Autodesk Fusion 360 part; units mm, degrees
(part 2 of 5)
  spline S268 degree 3 poles (57.7936, -18.906) (57.5187, -18.906) (57.2937, -18.681) (57.2937, -18.406) knots 0 0 0 0 1 1 1 1
  line L268 (57.2937, -18.406) -> (57.2937, -5.4062)
  spline S269 degree 3 poles (57.2937, -5.4062) (57.2937, -5.1311) (57.5187, -4.9062) (57.7936, -4.9062) knots 2 2 2 2 3 3 3 3
  line L269 (57.7936, -4.9062) -> (70.7933, -4.9062)
  spline S270 degree 3 poles (70.7933, -4.9062) (71.0686, -4.9062) (71.2935, -5.1311) (71.2935, -5.4062) knots 4 4 4 4 5 5 5 5
  line L270 (71.2935, -5.4062) -> (71.2935, -18.406)
  spline S271 degree 3 poles (71.2935, -18.406) (71.2935, -18.681) (71.0686, -18.906) (70.7933, -18.906) knots 6 6 6 6 7 7 7 7
  line L271 (70.7933, -18.906) -> (57.7936, -18.906)
  spline S272 degree 3 poles (-57.0067, -5.4062) (-57.0067, -5.1311) (-56.7818, -4.9062) (-56.5068, -4.9062) knots 0 0 0 0 1 1 1 1
  line L272 (-56.5068, -4.9062) -> (-43.5068, -4.9062)
  spline S273 degree 3 poles (-43.5068, -4.9062) (-43.2315, -4.9062) (-43.0065, -5.1311) (-43.0065, -5.4062) knots 2 2 2 2 3 3 3 3
  line L273 (-43.0065, -5.4062) -> (-43.0065, -18.406)
  spline S274 degree 3 poles (-43.0065, -18.406) (-43.0065, -18.681) (-43.2315, -18.906) (-43.5068, -18.906) knots 4 4 4 4 5 5 5 5
  line L274 (-43.5068, -18.906) -> (-56.5068, -18.906)
  spline S275 degree 3 poles (-56.5068, -18.906) (-56.7818, -18.906) (-57.0067, -18.681) (-57.0067, -18.406) knots 6 6 6 6 7 7 7 7
  line L275 (-57.0067, -18.406) -> (-57.0067, -5.4062)
  spline S276 degree 3 poles (129.2304, 0.144) (128.9555, 0.144) (128.7306, 0.369) (128.7306, 0.6441) knots 0 0 0 0 1 1 1 1
  line L276 (128.7306, 0.6441) -> (128.7306, 13.6438)
  spline S277 degree 3 poles (128.7306, 13.6438) (128.7306, 13.9189) (128.9555, 14.1438) (129.2304, 14.1438) knots 2 2 2 2 3 3 3 3
  line L277 (129.2304, 14.1438) -> (142.2305, 14.1438)
  spline S278 degree 3 poles (142.2305, 14.1438) (142.5058, 14.1438) (142.7307, 13.9189) (142.7307, 13.6438) knots 4 4 4 4 5 5 5 5
  line L278 (142.7307, 13.6438) -> (142.7307, 0.6441)
  spline S279 degree 3 poles (142.7307, 0.6441) (142.7307, 0.369) (142.5058, 0.144) (142.2305, 0.144) knots 6 6 6 6 7 7 7 7
  line L279 (142.2305, 0.144) -> (129.2304, 0.144)
  spline S280 degree 3 poles (76.8436, -18.906) (76.5687, -18.906) (76.3437, -18.681) (76.3437, -18.406) knots 0 0 0 0 1 1 1 1
  line L280 (76.3437, -18.406) -> (76.3437, -5.4062)
  spline S281 degree 3 poles (76.3437, -5.4062) (76.3437, -5.1311) (76.5687, -4.9062) (76.8436, -4.9062) knots 2 2 2 2 3 3 3 3
  line L281 (76.8436, -4.9062) -> (89.8433, -4.9062)
  spline S282 degree 3 poles (89.8433, -4.9062) (90.1186, -4.9062) (90.3436, -5.1311) (90.3436, -5.4062) knots 4 4 4 4 5 5 5 5
  line L282 (90.3436, -5.4062) -> (90.3436, -18.406)
  spline S283 degree 3 poles (90.3436, -18.406) (90.3436, -18.681) (90.1186, -18.906) (89.8433, -18.906) knots 6 6 6 6 7 7 7 7
  line L283 (89.8433, -18.906) -> (76.8436, -18.906)
  spline S284 degree 3 poles (23.9555, 32.6938) (23.9555, 32.9689) (24.1805, 33.1939) (24.4554, 33.1939) knots 0 0 0 0 1 1 1 1
  line L284 (24.4554, 33.1939) -> (37.4554, 33.1939)
  spline S285 degree 3 poles (37.4554, 33.1939) (37.7307, 33.1939) (37.9557, 32.9689) (37.9557, 32.6938) knots 2 2 2 2 3 3 3 3
  line L285 (37.9557, 32.6938) -> (37.9557, 19.6941)
  spline S286 degree 3 poles (37.9557, 19.6941) (37.9557, 19.419) (37.7307, 19.194) (37.4554, 19.194) knots 4 4 4 4 5 5 5 5
  line L286 (37.4554, 19.194) -> (24.4554, 19.194)
  spline S287 degree 3 poles (24.4554, 19.194) (24.1805, 19.194) (23.9555, 19.419) (23.9555, 19.6941) knots 6 6 6 6 7 7 7 7
  line L287 (23.9555, 19.6941) -> (23.9555, 32.6938)
  spline S288 degree 3 poles (95.3937, -5.4062) (95.3937, -5.1311) (95.6187, -4.9062) (95.8936, -4.9062) knots 0 0 0 0 1 1 1 1
  line L288 (95.8936, -4.9062) -> (108.8933, -4.9062)
  spline S289 degree 3 poles (108.8933, -4.9062) (109.1686, -4.9062) (109.3936, -5.1311) (109.3936, -5.4062) knots 2 2 2 2 3 3 3 3
  line L289 (109.3936, -5.4062) -> (109.3936, -18.406)
  spline S290 degree 3 poles (109.3936, -18.406) (109.3936, -18.681) (109.1686, -18.906) (108.8933, -18.906) knots 4 4 4 4 5 5 5 5
  line L290 (108.8933, -18.906) -> (95.8936, -18.906)
  spline S291 degree 3 poles (95.8936, -18.906) (95.6187, -18.906) (95.3937, -18.681) (95.3937, -18.406) knots 6 6 6 6 7 7 7 7
  line L291 (95.3937, -18.406) -> (95.3937, -5.4062)
  spline S292 degree 3 poles (38.7436, -18.906) (38.4687, -18.906) (38.2437, -18.681) (38.2437, -18.406) knots 0 0 0 0 1 1 1 1
  line L292 (38.2437, -18.406) -> (38.2437, -5.4062)
  spline S293 degree 3 poles (38.2437, -5.4062) (38.2437, -5.1311) (38.4687, -4.9062) (38.7436, -4.9062) knots 2 2 2 2 3 3 3 3
  line L293 (38.7436, -4.9062) -> (51.7433, -4.9062)
  spline S294 degree 3 poles (51.7433, -4.9062) (52.0186, -4.9062) (52.2435, -5.1311) (52.2435, -5.4062) knots 4 4 4 4 5 5 5 5
  line L294 (52.2435, -5.4062) -> (52.2435, -18.406)
  spline S295 degree 3 poles (52.2435, -18.406) (52.2435, -18.681) (52.0186, -18.906) (51.7433, -18.906) knots 6 6 6 6 7 7 7 7
  line L295 (51.7433, -18.906) -> (38.7436, -18.906)
  spline S296 degree 3 poles (-14.1445, 56.506) (-14.1445, 56.7811) (-13.9196, 57.006) (-13.6447, 57.006) knots 0 0 0 0 1 1 1 1
  line L296 (-13.6447, 57.006) -> (-0.6446, 57.006)
  spline S297 degree 3 poles (-0.6446, 57.006) (-0.3693, 57.006) (-0.1443, 56.7811) (-0.1443, 56.506) knots 2 2 2 2 3 3 3 3
  line L297 (-0.1443, 56.506) -> (-0.1443, 43.5059)
  spline S298 degree 3 poles (-0.1443, 43.5059) (-0.1443, 43.2308) (-0.3693, 43.0058) (-0.6446, 43.0058) knots 4 4 4 4 5 5 5 5
  line L298 (-0.6446, 43.0058) -> (-13.6447, 43.0058)
  spline S299 degree 3 poles (-13.6447, 43.0058) (-13.9196, 43.0058) (-14.1445, 43.2308) (-14.1445, 43.5059) knots 6 6 6 6 7 7 7 7
  line L299 (-14.1445, 43.5059) -> (-14.1445, 56.506)
  spline S300 degree 3 poles (91.1304, 0.144) (90.8555, 0.144) (90.6305, 0.369) (90.6305, 0.6441) knots 0 0 0 0 1 1 1 1
  line L300 (90.6305, 0.6441) -> (90.6305, 13.6438)
  spline S301 degree 3 poles (90.6305, 13.6438) (90.6305, 13.9189) (90.8555, 14.1438) (91.1304, 14.1438) knots 2 2 2 2 3 3 3 3
  line L301 (91.1304, 14.1438) -> (104.1305, 14.1438)
  spline S302 degree 3 poles (104.1305, 14.1438) (104.4058, 14.1438) (104.6307, 13.9189) (104.6307, 13.6438) knots 4 4 4 4 5 5 5 5
  line L302 (104.6307, 13.6438) -> (104.6307, 0.6441)
  spline S303 degree 3 poles (104.6307, 0.6441) (104.6307, 0.369) (104.4058, 0.144) (104.1305, 0.144) knots 6 6 6 6 7 7 7 7
  line L303 (104.1305, 0.144) -> (91.1304, 0.144)
  spline S304 degree 3 poles (-23.1697, 0.144) (-23.4446, 0.144) (-23.6695, 0.369) (-23.6695, 0.6441) knots 0 0 0 0 1 1 1 1
  line L304 (-23.6695, 0.6441) -> (-23.6695, 13.6438)
  spline S305 degree 3 poles (-23.6695, 13.6438) (-23.6695, 13.9189) (-23.4446, 14.1438) (-23.1697, 14.1438) knots 2 2 2 2 3 3 3 3
  line L305 (-23.1697, 14.1438) -> (-10.1696, 14.1438)
  spline S306 degree 3 poles (-10.1696, 14.1438) (-9.8943, 14.1438) (-9.6694, 13.9189) (-9.6694, 13.6438) knots 4 4 4 4 5 5 5 5
  line L306 (-9.6694, 13.6438) -> (-9.6694, 0.6441)
  spline S307 degree 3 poles (-9.6694, 0.6441) (-9.6694, 0.369) (-9.8943, 0.144) (-10.1696, 0.144) knots 6 6 6 6 7 7 7 7
  line L307 (-10.1696, 0.144) -> (-23.1697, 0.144)
  spline S308 degree 3 poles (-61.2697, 0.144) (-61.5446, 0.144) (-61.7696, 0.369) (-61.7696, 0.6441) knots 0 0 0 0 1 1 1 1
  line L308 (-61.7696, 0.6441) -> (-61.7696, 13.6438)
  spline S309 degree 3 poles (-61.7696, 13.6438) (-61.7696, 13.9189) (-61.5446, 14.1438) (-61.2697, 14.1438) knots 2 2 2 2 3 3 3 3
  line L309 (-61.2697, 14.1438) -> (-48.2696, 14.1438)
  spline S310 degree 3 poles (-48.2696, 14.1438) (-47.9943, 14.1438) (-47.7694, 13.9189) (-47.7694, 13.6438) knots 4 4 4 4 5 5 5 5
  line L310 (-47.7694, 13.6438) -> (-47.7694, 0.6441)
  spline S311 degree 3 poles (-47.7694, 0.6441) (-47.7694, 0.369) (-47.9943, 0.144) (-48.2696, 0.144) knots 6 6 6 6 7 7 7 7
  line L311 (-48.2696, 0.144) -> (-61.2697, 0.144)
  spline S312 degree 3 poles (119.2056, 32.6938) (119.2056, 32.9689) (119.4305, 33.1939) (119.7054, 33.1939) knots 0 0 0 0 1 1 1 1
  line L312 (119.7054, 33.1939) -> (132.7055, 33.1939)
  spline S313 degree 3 poles (132.7055, 33.1939) (132.9808, 33.1939) (133.2057, 32.9689) (133.2057, 32.6938) knots 2 2 2 2 3 3 3 3
  line L313 (133.2057, 32.6938) -> (133.2057, 19.6941)
  spline S314 degree 3 poles (133.2057, 19.6941) (133.2057, 19.419) (132.9808, 19.194) (132.7055, 19.194) knots 4 4 4 4 5 5 5 5
  line L314 (132.7055, 19.194) -> (119.7054, 19.194)
  spline S315 degree 3 poles (119.7054, 19.194) (119.4305, 19.194) (119.2056, 19.419) (119.2056, 19.6941) knots 6 6 6 6 7 7 7 7
  line L315 (119.2056, 19.6941) -> (119.2056, 32.6938)
  spline S316 degree 3 poles (4.9055, 32.6938) (4.9055, 32.9689) (5.1304, 33.1939) (5.4054, 33.1939) knots 0 0 0 0 1 1 1 1
  line L316 (5.4054, 33.1939) -> (18.4054, 33.1939)
  spline S317 degree 3 poles (18.4054, 33.1939) (18.6807, 33.1939) (18.9057, 32.9689) (18.9057, 32.6938) knots 2 2 2 2 3 3 3 3
  line L317 (18.9057, 32.6938) -> (18.9057, 19.6941)
  spline S318 degree 3 poles (18.9057, 19.6941) (18.9057, 19.419) (18.6807, 19.194) (18.4054, 19.194) knots 4 4 4 4 5 5 5 5
  line L318 (18.4054, 19.194) -> (5.4054, 19.194)
  spline S319 degree 3 poles (5.4054, 19.194) (5.1304, 19.194) (4.9055, 19.419) (4.9055, 19.6941) knots 6 6 6 6 7 7 7 7
  line L319 (4.9055, 19.6941) -> (4.9055, 32.6938)
  line L320 (71.5805, 0.6441) -> (71.5805, 13.6438)
  spline S320 degree 3 poles (71.5805, 13.6438) (71.5805, 13.9189) (71.8055, 14.1438) (72.0804, 14.1438) knots 1 1 1 1 2 2 2 2
  line L321 (72.0804, 14.1438) -> (85.0805, 14.1438)
  spline S321 degree 3 poles (85.0805, 14.1438) (85.3557, 14.1438) (85.5807, 13.9189) (85.5807, 13.6438) knots 3 3 3 3 4 4 4 4
  line L322 (85.5807, 13.6438) -> (85.5807, 0.6441)
  spline S322 degree 3 poles (85.5807, 0.6441) (85.5807, 0.369) (85.3557, 0.144) (85.0805, 0.144) knots 5 5 5 5 6 6 6 6
  line L323 (85.0805, 0.144) -> (72.0804, 0.144)
  spline S323 degree 3 poles (72.0804, 0.144) (71.8055, 0.144) (71.5805, 0.369) (71.5805, 0.6441) knots 7 7 7 7 8 8 8 8
  spline S324 degree 3 poles (81.1055, 56.506) (81.1055, 56.7811) (81.3305, 57.006) (81.6054, 57.006) knots 0 0 0 0 1 1 1 1
  line L324 (81.6054, 57.006) -> (94.6055, 57.006)
  spline S325 degree 3 poles (94.6055, 57.006) (94.8807, 57.006) (95.1057, 56.7811) (95.1057, 56.506) knots 2 2 2 2 3 3 3 3
  line L325 (95.1057, 56.506) -> (95.1057, 43.5059)
  spline S326 degree 3 poles (95.1057, 43.5059) (95.1057, 43.2308) (94.8807, 43.0058) (94.6055, 43.0058) knots 4 4 4 4 5 5 5 5
  line L326 (94.6055, 43.0058) -> (81.6054, 43.0058)
  spline S327 degree 3 poles (81.6054, 43.0058) (81.3305, 43.0058) (81.1055, 43.2308) (81.1055, 43.5059) knots 6 6 6 6 7 7 7 7
  line L327 (81.1055, 43.5059) -> (81.1055, 56.506)
  spline S328 degree 3 poles (66.8187, -24.4562) (66.8187, -24.1811) (67.0437, -23.9562) (67.3186, -23.9562) knots 0 0 0 0 1 1 1 1
  line L328 (67.3186, -23.9562) -> (80.3183, -23.9562)
  spline S329 degree 3 poles (80.3183, -23.9562) (80.5936, -23.9562) (80.8185, -24.1811) (80.8185, -24.4562) knots 2 2 2 2 3 3 3 3
  line L329 (80.8185, -24.4562) -> (80.8185, -37.456)
  spline S330 degree 3 poles (80.8185, -37.456) (80.8185, -37.7311) (80.5936, -37.956) (80.3183, -37.956) knots 4 4 4 4 5 5 5 5
  line L330 (80.3183, -37.956) -> (67.3186, -37.956)
  spline S331 degree 3 poles (67.3186, -37.956) (67.0437, -37.956) (66.8187, -37.7311) (66.8187, -37.456) knots 6 6 6 6 7 7 7 7
  line L331 (66.8187, -37.456) -> (66.8187, -24.4562)
  spline S332 degree 3 poles (9.6687, -24.4562) (9.6687, -24.1811) (9.8936, -23.9562) (10.1686, -23.9562) knots 0 0 0 0 1 1 1 1
  line L332 (10.1686, -23.9562) -> (23.1683, -23.9562)
  spline S333 degree 3 poles (23.1683, -23.9562) (23.4435, -23.9562) (23.6685, -24.1811) (23.6685, -24.4562) knots 2 2 2 2 3 3 3 3
  line L333 (23.6685, -24.4562) -> (23.6685, -37.456)
  spline S334 degree 3 poles (23.6685, -37.456) (23.6685, -37.7311) (23.4435, -37.956) (23.1683, -37.956) knots 4 4 4 4 5 5 5 5
  line L334 (23.1683, -37.956) -> (10.1686, -37.956)
  spline S335 degree 3 poles (10.1686, -37.956) (9.8936, -37.956) (9.6687, -37.7311) (9.6687, -37.456) knots 6 6 6 6 7 7 7 7
  line L335 (9.6687, -37.456) -> (9.6687, -24.4562)
  spline S336 degree 3 poles (62.0555, 32.6938) (62.0555, 32.9689) (62.2805, 33.1939) (62.5554, 33.1939) knots 0 0 0 0 1 1 1 1
  line L336 (62.5554, 33.1939) -> (75.5555, 33.1939)
  spline S337 degree 3 poles (75.5555, 33.1939) (75.8307, 33.1939) (76.0557, 32.9689) (76.0557, 32.6938) knots 2 2 2 2 3 3 3 3
  line L337 (76.0557, 32.6938) -> (76.0557, 19.6941)
  spline S338 degree 3 poles (76.0557, 19.6941) (76.0557, 19.419) (75.8307, 19.194) (75.5555, 19.194) knots 4 4 4 4 5 5 5 5
  line L338 (75.5555, 19.194) -> (62.5554, 19.194)
  spline S339 degree 3 poles (62.5554, 19.194) (62.2805, 19.194) (62.0555, 19.419) (62.0555, 19.6941) knots 6 6 6 6 7 7 7 7
  line L339 (62.0555, 19.6941) -> (62.0555, 32.6938)
  spline S340 degree 3 poles (43.0055, 56.506) (43.0055, 56.7811) (43.2305, 57.006) (43.5054, 57.006) knots 0 0 0 0 1 1 1 1
  line L340 (43.5054, 57.006) -> (56.5055, 57.006)
  spline S341 degree 3 poles (56.5055, 57.006) (56.7807, 57.006) (57.0057, 56.7811) (57.0057, 56.506) knots 2 2 2 2 3 3 3 3
  line L341 (57.0057, 56.506) -> (57.0057, 43.5059)
  spline S342 degree 3 poles (57.0057, 43.5059) (57.0057, 43.2308) (56.7807, 43.0058) (56.5055, 43.0058) knots 4 4 4 4 5 5 5 5
  line L342 (56.5055, 43.0058) -> (43.5054, 43.0058)
  spline S343 degree 3 poles (43.5054, 43.0058) (43.2305, 43.0058) (43.0055, 43.2308) (43.0055, 43.5059) knots 6 6 6 6 7 7 7 7
  line L343 (43.0055, 43.5059) -> (43.0055, 56.506)
  spline S344 degree 3 poles (-52.2446, 32.6938) (-52.2446, 32.9689) (-52.0196, 33.1939) (-51.7447, 33.1939) knots 0 0 0 0 1 1 1 1
  line L344 (-51.7447, 33.1939) -> (-38.7446, 33.1939)
  spline S345 degree 3 poles (-38.7446, 33.1939) (-38.4693, 33.1939) (-38.2444, 32.9689) (-38.2444, 32.6938) knots 2 2 2 2 3 3 3 3
  line L345 (-38.2444, 32.6938) -> (-38.2444, 19.6941)
  spline S346 degree 3 poles (-38.2444, 19.6941) (-38.2444, 19.419) (-38.4693, 19.194) (-38.7446, 19.194) knots 4 4 4 4 5 5 5 5
  line L346 (-38.7446, 19.194) -> (-51.7447, 19.194)
  spline S347 degree 3 poles (-51.7447, 19.194) (-52.0196, 19.194) (-52.2446, 19.419) (-52.2446, 19.6941) knots 6 6 6 6 7 7 7 7
  line L347 (-52.2446, 19.6941) -> (-52.2446, 32.6938)
  spline S348 degree 3 poles (81.1055, 32.6938) (81.1055, 32.9689) (81.3305, 33.1939) (81.6054, 33.1939) knots 0 0 0 0 1 1 1 1
  line L348 (81.6054, 33.1939) -> (94.6055, 33.1939)
  spline S349 degree 3 poles (94.6055, 33.1939) (94.8807, 33.1939) (95.1057, 32.9689) (95.1057, 32.6938) knots 2 2 2 2 3 3 3 3
  line L349 (95.1057, 32.6938) -> (95.1057, 19.6941)
  spline S350 degree 3 poles (95.1057, 19.6941) (95.1057, 19.419) (94.8807, 19.194) (94.6055, 19.194) knots 4 4 4 4 5 5 5 5
  line L350 (94.6055, 19.194) -> (81.6054, 19.194)
  spline S351 degree 3 poles (81.6054, 19.194) (81.3305, 19.194) (81.1055, 19.419) (81.1055, 19.6941) knots 6 6 6 6 7 7 7 7
  line L351 (81.1055, 19.6941) -> (81.1055, 32.6938)
  spline S352 degree 3 poles (-100.1566, -56.506) (-100.1566, -56.7811) (-100.3815, -57.006) (-100.6568, -57.006) knots 0 0 0 0 1 1 1 1
  line L352 (-100.6568, -57.006) -> (-113.6569, -57.006)
  spline S353 degree 3 poles (-113.6569, -57.006) (-113.9318, -57.006) (-114.1568, -56.7811) (-114.1568, -56.506) knots 2 2 2 2 3 3 3 3
  line L353 (-114.1568, -56.506) -> (-114.1568, -43.5062)
  spline S354 degree 3 poles (-114.1568, -43.5062) (-114.1568, -43.2312) (-113.9318, -43.0062) (-113.6569, -43.0062) knots 4 4 4 4 5 5 5 5
  line L354 (-113.6569, -43.0062) -> (-100.6568, -43.0062)
  spline S355 degree 3 poles (-100.6568, -43.0062) (-100.3815, -43.0062) (-100.1566, -43.2312) (-100.1566, -43.5062) knots 6 6 6 6 7 7 7 7
  line L355 (-100.1566, -43.5062) -> (-100.1566, -56.506)
  spline S356 degree 3 poles (99.8686, -37.456) (99.8686, -37.7311) (99.6436, -37.956) (99.3683, -37.956) knots 0 0 0 0 1 1 1 1
  line L356 (99.3683, -37.956) -> (86.3686, -37.956)
  spline S357 degree 3 poles (86.3686, -37.956) (86.0937, -37.956) (85.8687, -37.7311) (85.8687, -37.456) knots 2 2 2 2 3 3 3 3
  line L357 (85.8687, -37.456) -> (85.8687, -24.4562)
  spline S358 degree 3 poles (85.8687, -24.4562) (85.8687, -24.1811) (86.0937, -23.9562) (86.3686, -23.9562) knots 4 4 4 4 5 5 5 5
  line L358 (86.3686, -23.9562) -> (99.3683, -23.9562)
  spline S359 degree 3 poles (99.3683, -23.9562) (99.6436, -23.9562) (99.8686, -24.1811) (99.8686, -24.4562) knots 6 6 6 6 7 7 7 7
  line L359 (99.8686, -24.4562) -> (99.8686, -37.456)
  spline S360 degree 3 poles (-55.3386, -30.9561) (-55.3386, -31.2312) (-55.4681, -31.4562) (-55.6263, -31.4562) (-55.7847, -31.4562) (-55.9143, -31.6811) (-55.9143, -31.9562) knots 0 0 0 0 1 1 1 2 2 2 2
  line L360 (-55.9143, -31.9562) -> (-55.9143, -37.2262)
  spline S361 degree 3 poles (-55.9143, -37.2262) (-55.9143, -37.5013) (-56.1392, -37.7262) (-56.4142, -37.7262) knots 3 3 3 3 4 4 4 4
  line L361 (-56.4142, -37.7262) -> (-57.139, -37.7262)
  spline S362 degree 3 poles (-57.139, -37.7262) (-57.4143, -37.7262) (-57.6392, -37.9512) (-57.6392, -38.2263) knots 5 5 5 5 6 6 6 6
  line L362 (-57.6392, -38.2263) -> (-57.6392, -38.4261)
  spline S363 degree 3 poles (-57.6392, -38.4261) (-57.6392, -38.7012) (-57.8642, -38.9262) (-58.1391, -38.9262) knots 7 7 7 7 8 8 8 8
  line L363 (-58.1391, -38.9262) -> (-60.7891, -38.9262)
  spline S364 degree 3 poles (-60.7891, -38.9262) (-61.064, -38.9262) (-61.289, -38.7012) (-61.289, -38.4261) knots 9 9 9 9 10 10 10 10
  line L364 (-61.289, -38.4261) -> (-61.289, -38.2263)
  spline S365 degree 3 poles (-61.289, -38.2263) (-61.289, -37.9512) (-61.5139, -37.7262) (-61.7892, -37.7262) knots 11 11 11 11 12 12 12 12
  line L365 (-61.7892, -37.7262) -> (-62.5141, -37.7262)
  spline S366 degree 3 poles (-62.5141, -37.7262) (-62.7893, -37.7262) (-63.0143, -37.5013) (-63.0143, -37.2262) knots 13 13 13 13 14 14 14 14
  line L366 (-63.0143, -37.2262) -> (-63.0143, -33.7563)
  spline S367 degree 3 poles (-63.0143, -33.7563) (-63.0143, -33.4812) (-63.2392, -33.2562) (-63.5142, -33.2562) knots 15 15 15 15 16 16 16 16
  line L367 (-63.5142, -33.2562) -> (-63.9386, -33.2562)
  spline S368 degree 3 poles (-63.9386, -33.2562) (-64.2135, -33.2562) (-64.4385, -33.4812) (-64.4385, -33.7563) knots 17 17 17 17 18 18 18 18
  line L368 (-64.4385, -33.7563) -> (-64.4385, -37.456)
  spline S369 degree 3 poles (-64.4385, -37.456) (-64.4385, -37.7311) (-64.6635, -37.956) (-64.9387, -37.956) knots 19 19 19 19 20 20 20 20
  line L369 (-64.9387, -37.956) -> (-77.9388, -37.956)
  spline S370 degree 3 poles (-77.9388, -37.956) (-78.2137, -37.956) (-78.4387, -37.7311) (-78.4387, -37.456) knots 21 21 21 21 22 22 22 22
  line L370 (-78.4387, -37.456) -> (-78.4387, -33.7563)
  spline S371 degree 3 poles (-78.4387, -33.7563) (-78.4387, -33.4812) (-78.6636, -33.2562) (-78.9389, -33.2562) knots 23 23 23 23 24 24 24 24
  line L371 (-78.9389, -33.2562) -> (-79.363, -33.2562)
  spline S372 degree 3 poles (-79.363, -33.2562) (-79.6383, -33.2562) (-79.8632, -33.4812) (-79.8632, -33.7563) knots 25 25 25 25 26 26 26 26
  line L372 (-79.8632, -33.7563) -> (-79.8632, -37.2262)
  spline S373 degree 3 poles (-79.8632, -37.2262) (-79.8632, -37.5013) (-80.0882, -37.7262) (-80.3631, -37.7262) knots 27 27 27 27 28 28 28 28
  line L373 (-80.3631, -37.7262) -> (-81.089, -37.7262)
  spline S374 degree 3 poles (-81.089, -37.7262) (-81.3643, -37.7262) (-81.5892, -37.9512) (-81.5892, -38.2263) knots 29 29 29 29 30 30 30 30
  line L374 (-81.5892, -38.2263) -> (-81.5892, -38.4261)
  spline S375 degree 3 poles (-81.5892, -38.4261) (-81.5892, -38.7012) (-81.8142, -38.9262) (-82.0891, -38.9262) knots 31 31 31 31 32 32 32 32
  line L375 (-82.0891, -38.9262) -> (-84.738, -38.9262)
  spline S376 degree 3 poles (-84.738, -38.9262) (-85.0133, -38.9262) (-85.2383, -38.7012) (-85.2383, -38.4261) knots 33 33 33 33 34 34 34 34
  line L376 (-85.2383, -38.4261) -> (-85.2383, -38.2263)
  spline S377 degree 3 poles (-85.2383, -38.2263) (-85.2383, -37.9512) (-85.4632, -37.7262) (-85.7381, -37.7262) knots 35 35 35 35 36 36 36 36
  line L377 (-85.7381, -37.7262) -> (-86.463, -37.7262)
  spline S378 degree 3 poles (-86.463, -37.7262) (-86.7383, -37.7262) (-86.9632, -37.5013) (-86.9632, -37.2262) knots 37 37 37 37 38 38 38 38
  line L378 (-86.9632, -37.2262) -> (-86.9632, -31.9562)
  spline S379 degree 3 poles (-86.9632, -31.9562) (-86.9632, -31.6811) (-87.0928, -31.4562) (-87.409, -31.4562) (-87.5386, -31.2312) (-87.5386, -30.9561) knots 39 39 39 39 40 40 41 41 41 41
  line L379 (-87.5386, -30.9561) -> (-87.5386, -29.156)
  spline S380 degree 3 poles (-87.5386, -29.156) (-87.5386, -28.8809) (-87.409, -28.656) (-87.0928, -28.656) (-86.9632, -28.431) (-86.9632, -28.1559) knots 42 42 42 42 43 43 44 44 44 44
  line L380 (-86.9632, -28.1559) -> (-86.9632, -25.426)
  spline S381 degree 3 poles (-86.9632, -25.426) (-86.9632, -25.1509) (-86.7383, -24.926) (-86.463, -24.926) knots 45 45 45 45 46 46 46 46
  line L381 (-86.463, -24.926) -> (-80.3631, -24.926)
  spline S382 degree 3 poles (-80.3631, -24.926) (-80.0882, -24.926) (-79.8632, -25.1509) (-79.8632, -25.426) knots 47 47 47 47 48 48 48 48
  line L382 (-79.8632, -25.426) -> (-79.8632, -28.1559)
  spline S383 degree 3 poles (-79.8632, -28.1559) (-79.8632, -28.431) (-79.6383, -28.656) (-79.363, -28.656) knots 49 49 49 49 50 50 50 50
  line L383 (-79.363, -28.656) -> (-78.9389, -28.656)
  spline S384 degree 3 poles (-78.9389, -28.656) (-78.6636, -28.656) (-78.4387, -28.431) (-78.4387, -28.1559) knots 51 51 51 51 52 52 52 52
  line L384 (-78.4387, -28.1559) -> (-78.4387, -24.4562)
  spline S385 degree 3 poles (-78.4387, -24.4562) (-78.4387, -24.1811) (-78.2137, -23.9562) (-77.9388, -23.9562) knots 53 53 53 53 54 54 54 54
  line L385 (-77.9388, -23.9562) -> (-64.9387, -23.9562)
  spline S386 degree 3 poles (-64.9387, -23.9562) (-64.6635, -23.9562) (-64.4385, -24.1811) (-64.4385, -24.4562) knots 55 55 55 55 56 56 56 56
  line L386 (-64.4385, -24.4562) -> (-64.4385, -28.1559)
  spline S387 degree 3 poles (-64.4385, -28.1559) (-64.4385, -28.431) (-64.2135, -28.656) (-63.9386, -28.656) knots 57 57 57 57 58 58 58 58
  line L387 (-63.9386, -28.656) -> (-63.5142, -28.656)
  spline S388 degree 3 poles (-63.5142, -28.656) (-63.2392, -28.656) (-63.0143, -28.431) (-63.0143, -28.1559) knots 59 59 59 59 60 60 60 60
  line L388 (-63.0143, -28.1559) -> (-63.0143, -25.426)
  spline S389 degree 3 poles (-63.0143, -25.426) (-63.0143, -25.1509) (-62.7893, -24.926) (-62.5141, -24.926) knots 61 61 61 61 62 62 62 62
  line L389 (-62.5141, -24.926) -> (-56.4142, -24.926)
  spline S390 degree 3 poles (-56.4142, -24.926) (-56.1392, -24.926) (-55.9143, -25.1509) (-55.9143, -25.426) knots 63 63 63 63 64 64 64 64
  line L390 (-55.9143, -25.426) -> (-55.9143, -28.1559)
  spline S391 degree 3 poles (-55.9143, -28.1559) (-55.9143, -28.431) (-55.7847, -28.656) (-55.6263, -28.656) (-55.4681, -28.656) (-55.3386, -28.8809) (-55.3386, -29.156) knots 65 65 65 65 66 66 66 67 67 67 67
  line L391 (-55.3386, -29.156) -> (-55.3386, -30.9561)
  spline S392 degree 3 poles (-76.3447, -56.506) (-76.3447, -56.7811) (-76.5697, -57.006) (-76.845, -57.006) knots 0 0 0 0 1 1 1 1
  line L392 (-76.845, -57.006) -> (-89.8447, -57.006)
  spline S393 degree 3 poles (-89.8447, -57.006) (-90.1196, -57.006) (-90.3446, -56.7811) (-90.3446, -56.506) knots 2 2 2 2 3 3 3 3
  line L393 (-90.3446, -56.506) -> (-90.3446, -43.5062)
  spline S394 degree 3 poles (-90.3446, -43.5062) (-90.3446, -43.2312) (-90.1196, -43.0062) (-89.8447, -43.0062) knots 4 4 4 4 5 5 5 5
  line L394 (-89.8447, -43.0062) -> (-76.845, -43.0062)
  spline S395 degree 3 poles (-76.845, -43.0062) (-76.5697, -43.0062) (-76.3447, -43.2312) (-76.3447, -43.5062) knots 6 6 6 6 7 7 7 7
  line L395 (-76.3447, -43.5062) -> (-76.3447, -56.506)
  spline S396 degree 3 poles (-138.2566, -56.506) (-138.2566, -56.7811) (-138.4816, -57.006) (-138.7568, -57.006) knots 0 0 0 0 1 1 1 1
  line L396 (-138.7568, -57.006) -> (-151.7569, -57.006)
  spline S397 degree 3 poles (-151.7569, -57.006) (-152.0318, -57.006) (-152.2568, -56.7811) (-152.2568, -56.506) knots 2 2 2 2 3 3 3 3
  line L397 (-152.2568, -56.506) -> (-152.2568, -43.5062)
  spline S398 degree 3 poles (-152.2568, -43.5062) (-152.2568, -43.2312) (-152.0318, -43.0062) (-151.7569, -43.0062) knots 4 4 4 4 5 5 5 5
  line L398 (-151.7569, -43.0062) -> (-138.7568, -43.0062)
  spline S399 degree 3 poles (-138.7568, -43.0062) (-138.4816, -43.0062) (-138.2566, -43.2312) (-138.2566, -43.5062) knots 6 6 6 6 7 7 7 7
  line L399 (-138.2566, -43.5062) -> (-138.2566, -56.506)
  spline S400 degree 3 poles (-100.1566, -18.406) (-100.1566, -18.681) (-100.3815, -18.906) (-100.6568, -18.906) knots 0 0 0 0 1 1 1 1
  line L400 (-100.6568, -18.906) -> (-113.6569, -18.906)
  spline S401 degree 3 poles (-113.6569, -18.906) (-113.9318, -18.906) (-114.1568, -18.681) (-114.1568, -18.406) knots 2 2 2 2 3 3 3 3
  line L401 (-114.1568, -18.406) -> (-114.1568, -5.4062)
  spline S402 degree 3 poles (-114.1568, -5.4062) (-114.1568, -5.1311) (-113.9318, -4.9062) (-113.6569, -4.9062) knots 4 4 4 4 5 5 5 5
  line L402 (-113.6569, -4.9062) -> (-100.6568, -4.9062)
  spline S403 degree 3 poles (-100.6568, -4.9062) (-100.3815, -4.9062) (-100.1566, -5.1311) (-100.1566, -5.4062) knots 6 6 6 6 7 7 7 7
  line L403 (-100.1566, -5.4062) -> (-100.1566, -18.406)
  spline S404 degree 3 poles (114.1557, -56.506) (114.1557, -56.7811) (113.9308, -57.006) (113.6555, -57.006) knots 0 0 0 0 1 1 1 1
  line L404 (113.6555, -57.006) -> (100.6554, -57.006)
  spline S405 degree 3 poles (100.6554, -57.006) (100.3805, -57.006) (100.1555, -56.7811) (100.1555, -56.506) knots 2 2 2 2 3 3 3 3
  line L405 (100.1555, -56.506) -> (100.1555, -43.5062)
  spline S406 degree 3 poles (100.1555, -43.5062) (100.1555, -43.2312) (100.3805, -43.0062) (100.6554, -43.0062) knots 4 4 4 4 5 5 5 5
  line L406 (100.6554, -43.0062) -> (113.6555, -43.0062)
  spline S407 degree 3 poles (113.6555, -43.0062) (113.9308, -43.0062) (114.1557, -43.2312) (114.1557, -43.5062) knots 6 6 6 6 7 7 7 7
  line L407 (114.1557, -43.5062) -> (114.1557, -56.506)
  spline S408 degree 3 poles (-38.2444, -56.506) (-38.2444, -56.7811) (-38.4693, -57.006) (-38.7446, -57.006) knots 0 0 0 0 1 1 1 1
  line L408 (-38.7446, -57.006) -> (-51.7447, -57.006)
  spline S409 degree 3 poles (-51.7447, -57.006) (-52.0196, -57.006) (-52.2446, -56.7811) (-52.2446, -56.506) knots 2 2 2 2 3 3 3 3
  line L409 (-52.2446, -56.506) -> (-52.2446, -43.5062)
  spline S410 degree 3 poles (-52.2446, -43.5062) (-52.2446, -43.2312) (-52.0196, -43.0062) (-51.7447, -43.0062) knots 4 4 4 4 5 5 5 5
  line L410 (-51.7447, -43.0062) -> (-38.7446, -43.0062)
  spline S411 degree 3 poles (-38.7446, -43.0062) (-38.4693, -43.0062) (-38.2444, -43.2312) (-38.2444, -43.5062) knots 6 6 6 6 7 7 7 7
  line L411 (-38.2444, -43.5062) -> (-38.2444, -56.506)
  spline S412 degree 3 poles (-138.2566, -18.406) (-138.2566, -18.681) (-138.4816, -18.906) (-138.7568, -18.906) knots 0 0 0 0 1 1 1 1
  line L412 (-138.7568, -18.906) -> (-151.7569, -18.906)
  spline S413 degree 3 poles (-151.7569, -18.906) (-152.0318, -18.906) (-152.2568, -18.681) (-152.2568, -18.406) knots 2 2 2 2 3 3 3 3
  line L413 (-152.2568, -18.406) -> (-152.2568, -5.4062)
  spline S414 degree 3 poles (-152.2568, -5.4062) (-152.2568, -5.1311) (-152.0318, -4.9062) (-151.7569, -4.9062) knots 4 4 4 4 5 5 5 5
  line L414 (-151.7569, -4.9062) -> (-138.7568, -4.9062)
  spline S415 degree 3 poles (-138.7568, -4.9062) (-138.4816, -4.9062) (-138.2566, -5.1311) (-138.2566, -5.4062) knots 6 6 6 6 7 7 7 7
  line L415 (-138.2566, -5.4062) -> (-138.2566, -18.406)
  spline S416 degree 3 poles (-100.1566, -37.456) (-100.1566, -37.7311) (-100.3815, -37.956) (-100.6568, -37.956) knots 0 0 0 0 1 1 1 1
  line L416 (-100.6568, -37.956) -> (-113.6569, -37.956)
  spline S417 degree 3 poles (-113.6569, -37.956) (-113.9318, -37.956) (-114.1568, -37.7311) (-114.1568, -37.456) knots 2 2 2 2 3 3 3 3
  line L417 (-114.1568, -37.456) -> (-114.1568, -24.4562)
  spline S418 degree 3 poles (-114.1568, -24.4562) (-114.1568, -24.1811) (-113.9318, -23.9562) (-113.6569, -23.9562) knots 4 4 4 4 5 5 5 5
  line L418 (-113.6569, -23.9562) -> (-100.6568, -23.9562)
  spline S419 degree 3 poles (-100.6568, -23.9562) (-100.3815, -23.9562) (-100.1566, -24.1811) (-100.1566, -24.4562) knots 6 6 6 6 7 7 7 7
  line L419 (-100.1566, -24.4562) -> (-100.1566, -37.456)
  spline S420 degree 3 poles (-119.2066, -18.406) (-119.2066, -18.681) (-119.4315, -18.906) (-119.7068, -18.906) knots 0 0 0 0 1 1 1 1
  line L420 (-119.7068, -18.906) -> (-132.7069, -18.906)
  spline S421 degree 3 poles (-132.7069, -18.906) (-132.9818, -18.906) (-133.2068, -18.681) (-133.2068, -18.406) knots 2 2 2 2 3 3 3 3
  line L421 (-133.2068, -18.406) -> (-133.2068, -5.4062)
  spline S422 degree 3 poles (-133.2068, -5.4062) (-133.2068, -5.1311) (-132.9818, -4.9062) (-132.7069, -4.9062) knots 4 4 4 4 5 5 5 5
  line L422 (-132.7069, -4.9062) -> (-119.7068, -4.9062)
  spline S423 degree 3 poles (-119.7068, -4.9062) (-119.4315, -4.9062) (-119.2066, -5.1311) (-119.2066, -5.4062) knots 6 6 6 6 7 7 7 7
  line L423 (-119.2066, -5.4062) -> (-119.2066, -18.406)
  spline S424 degree 3 poles (-138.2566, 0.6441) (-138.2566, 0.369) (-138.4816, 0.144) (-138.7568, 0.144) knots 0 0 0 0 1 1 1 1
  line L424 (-138.7568, 0.144) -> (-151.7569, 0.144)
  spline S425 degree 3 poles (-151.7569, 0.144) (-152.0318, 0.144) (-152.2568, 0.369) (-152.2568, 0.6441) knots 2 2 2 2 3 3 3 3
  line L425 (-152.2568, 0.6441) -> (-152.2568, 13.6438)
  spline S426 degree 3 poles (-152.2568, 13.6438) (-152.2568, 13.9189) (-152.0318, 14.1438) (-151.7569, 14.1438) knots 4 4 4 4 5 5 5 5
  line L426 (-151.7569, 14.1438) -> (-138.7568, 14.1438)
  spline S427 degree 3 poles (-138.7568, 14.1438) (-138.4816, 14.1438) (-138.2566, 13.9189) (-138.2566, 13.6438) knots 6 6 6 6 7 7 7 7
  line L427 (-138.2566, 13.6438) -> (-138.2566, 0.6441)
  spline S428 degree 3 poles (-100.1566, 0.6441) (-100.1566, 0.369) (-100.3815, 0.144) (-100.6568, 0.144) knots 0 0 0 0 1 1 1 1
  line L428 (-100.6568, 0.144) -> (-113.6569, 0.144)
  spline S429 degree 3 poles (-113.6569, 0.144) (-113.9318, 0.144) (-114.1568, 0.369) (-114.1568, 0.6441) knots 2 2 2 2 3 3 3 3
  line L429 (-114.1568, 0.6441) -> (-114.1568, 13.6438)
  spline S430 degree 3 poles (-114.1568, 13.6438) (-114.1568, 13.9189) (-113.9318, 14.1438) (-113.6569, 14.1438) knots 4 4 4 4 5 5 5 5
  line L430 (-113.6569, 14.1438) -> (-100.6568, 14.1438)
  spline S431 degree 3 poles (-100.6568, 14.1438) (-100.3815, 14.1438) (-100.1566, 13.9189) (-100.1566, 13.6438) knots 6 6 6 6 7 7 7 7
  line L431 (-100.1566, 13.6438) -> (-100.1566, 0.6441)
  spline S432 degree 3 poles (-119.2066, 43.5059) (-119.2066, 43.2308) (-119.4315, 43.0058) (-119.7068, 43.0058) knots 0 0 0 0 1 1 1 1
  line L432 (-119.7068, 43.0058) -> (-132.7069, 43.0058)
  spline S433 degree 3 poles (-132.7069, 43.0058) (-132.9818, 43.0058) (-133.2068, 43.2308) (-133.2068, 43.5059) knots 2 2 2 2 3 3 3 3
  line L433 (-133.2068, 43.5059) -> (-133.2068, 56.506)
  spline S434 degree 3 poles (-133.2068, 56.506) (-133.2068, 56.7811) (-132.9818, 57.006) (-132.7069, 57.006) knots 4 4 4 4 5 5 5 5
  line L434 (-132.7069, 57.006) -> (-119.7068, 57.006)
  spline S435 degree 3 poles (-119.7068, 57.006) (-119.4315, 57.006) (-119.2066, 56.7811) (-119.2066, 56.506) knots 6 6 6 6 7 7 7 7
  line L435 (-119.2066, 56.506) -> (-119.2066, 43.5059)
  spline S436 degree 3 poles (-100.1566, 24.4559) (-100.1566, 24.1808) (-100.3815, 23.9558) (-100.6568, 23.9558) knots 0 0 0 0 1 1 1 1
  line L436 (-100.6568, 23.9558) -> (-113.6569, 23.9558)
  spline S437 degree 3 poles (-113.6569, 23.9558) (-113.9318, 23.9558) (-114.1568, 24.1808) (-114.1568, 24.4559) knots 2 2 2 2 3 3 3 3
  line L437 (-114.1568, 24.4559) -> (-114.1568, 37.456)
  spline S438 degree 3 poles (-114.1568, 37.456) (-114.1568, 37.7311) (-113.9318, 37.956) (-113.6569, 37.956) knots 4 4 4 4 5 5 5 5
  line L438 (-113.6569, 37.956) -> (-100.6568, 37.956)
  spline S439 degree 3 poles (-100.6568, 37.956) (-100.3815, 37.956) (-100.1566, 37.7311) (-100.1566, 37.456) knots 6 6 6 6 7 7 7 7
  line L439 (-100.1566, 37.456) -> (-100.1566, 24.4559)
  spline S440 degree 3 poles (-119.2066, -37.456) (-119.2066, -37.7311) (-119.4315, -37.956) (-119.7068, -37.956) knots 0 0 0 0 1 1 1 1
  line L440 (-119.7068, -37.956) -> (-132.7069, -37.956)
  spline S441 degree 3 poles (-132.7069, -37.956) (-132.9818, -37.956) (-133.2068, -37.7311) (-133.2068, -37.456) knots 2 2 2 2 3 3 3 3
  line L441 (-133.2068, -37.456) -> (-133.2068, -24.4562)
  spline S442 degree 3 poles (-133.2068, -24.4562) (-133.2068, -24.1811) (-132.9818, -23.9562) (-132.7069, -23.9562) knots 4 4 4 4 5 5 5 5
  line L442 (-132.7069, -23.9562) -> (-119.7068, -23.9562)
  spline S443 degree 3 poles (-119.7068, -23.9562) (-119.4315, -23.9562) (-119.2066, -24.1811) (-119.2066, -24.4562) knots 6 6 6 6 7 7 7 7
  line L443 (-119.2066, -24.4562) -> (-119.2066, -37.456)
  spline S444 degree 3 poles (-100.1566, 43.5059) (-100.1566, 43.2308) (-100.3815, 43.0058) (-100.6568, 43.0058) knots 0 0 0 0 1 1 1 1
  line L444 (-100.6568, 43.0058) -> (-113.6569, 43.0058)
  spline S445 degree 3 poles (-113.6569, 43.0058) (-113.9318, 43.0058) (-114.1568, 43.2308) (-114.1568, 43.5059) knots 2 2 2 2 3 3 3 3
  line L445 (-114.1568, 43.5059) -> (-114.1568, 56.506)
  spline S446 degree 3 poles (-114.1568, 56.506) (-114.1568, 56.7811) (-113.9318, 57.006) (-113.6569, 57.006) knots 4 4 4 4 5 5 5 5
  line L446 (-113.6569, 57.006) -> (-100.6568, 57.006)
  spline S447 degree 3 poles (-100.6568, 57.006) (-100.3815, 57.006) (-100.1566, 56.7811) (-100.1566, 56.506) knots 6 6 6 6 7 7 7 7
  line L447 (-100.1566, 56.506) -> (-100.1566, 43.5059)
  spline S448 degree 3 poles (-119.2066, -56.506) (-119.2066, -56.7811) (-119.4315, -57.006) (-119.7068, -57.006) knots 0 0 0 0 1 1 1 1
  line L448 (-119.7068, -57.006) -> (-132.7069, -57.006)
  spline S449 degree 3 poles (-132.7069, -57.006) (-132.9818, -57.006) (-133.2068, -56.7811) (-133.2068, -56.506) knots 2 2 2 2 3 3 3 3
  line L449 (-133.2068, -56.506) -> (-133.2068, -43.5062)
  spline S450 degree 3 poles (-133.2068, -43.5062) (-133.2068, -43.2312) (-132.9818, -43.0062) (-132.7069, -43.0062) knots 4 4 4 4 5 5 5 5
  line L450 (-132.7069, -43.0062) -> (-119.7068, -43.0062)
  spline S451 degree 3 poles (-119.7068, -43.0062) (-119.4315, -43.0062) (-119.2066, -43.2312) (-119.2066, -43.5062) knots 6 6 6 6 7 7 7 7
  line L451 (-119.2066, -43.5062) -> (-119.2066, -56.506)
  spline S452 degree 3 poles (-157.3066, 24.4559) (-157.3066, 24.1808) (-157.5316, 23.9558) (-157.8068, 23.9558) knots 0 0 0 0 1 1 1 1
  line L452 (-157.8068, 23.9558) -> (-170.8069, 23.9558)
  spline S453 degree 3 poles (-170.8069, 23.9558) (-171.0818, 23.9558) (-171.3068, 24.1808) (-171.3068, 24.4559) knots 2 2 2 2 3 3 3 3
  line L453 (-171.3068, 24.4559) -> (-171.3068, 37.456)
  spline S454 degree 3 poles (-171.3068, 37.456) (-171.3068, 37.7311) (-171.0818, 37.956) (-170.8069, 37.956) knots 4 4 4 4 5 5 5 5
  line L454 (-170.8069, 37.956) -> (-157.8068, 37.956)
  spline S455 degree 3 poles (-157.8068, 37.956) (-157.5316, 37.956) (-157.3066, 37.7311) (-157.3066, 37.456) knots 6 6 6 6 7 7 7 7
  line L455 (-157.3066, 37.456) -> (-157.3066, 24.4559)
  spline S456 degree 3 poles (-119.2066, 0.6441) (-119.2066, 0.369) (-119.4315, 0.144) (-119.7068, 0.144) knots 0 0 0 0 1 1 1 1
  line L456 (-119.7068, 0.144) -> (-132.7069, 0.144)
  spline S457 degree 3 poles (-132.7069, 0.144) (-132.9818, 0.144) (-133.2068, 0.369) (-133.2068, 0.6441) knots 2 2 2 2 3 3 3 3
  line L457 (-133.2068, 0.6441) -> (-133.2068, 13.6438)
  spline S458 degree 3 poles (-133.2068, 13.6438) (-133.2068, 13.9189) (-132.9818, 14.1438) (-132.7069, 14.1438) knots 4 4 4 4 5 5 5 5
  line L458 (-132.7069, 14.1438) -> (-119.7068, 14.1438)
  spline S459 degree 3 poles (-119.7068, 14.1438) (-119.4315, 14.1438) (-119.2066, 13.9189) (-119.2066, 13.6438) knots 6 6 6 6 7 7 7 7
  line L459 (-119.2066, 13.6438) -> (-119.2066, 0.6441)
  spline S460 degree 3 poles (-33.4815, -37.456) (-33.4815, -37.7311) (-33.7065, -37.956) (-33.9818, -37.956) knots 0 0 0 0 1 1 1 1
  line L460 (-33.9818, -37.956) -> (-46.9815, -37.956)
  spline S461 degree 3 poles (-46.9815, -37.956) (-47.2564, -37.956) (-47.4814, -37.7311) (-47.4814, -37.456) knots 2 2 2 2 3 3 3 3
  line L461 (-47.4814, -37.456) -> (-47.4814, -24.4562)
  spline S462 degree 3 poles (-47.4814, -24.4562) (-47.4814, -24.1811) (-47.2564, -23.9562) (-46.9815, -23.9562) knots 4 4 4 4 5 5 5 5
  line L462 (-46.9815, -23.9562) -> (-33.9818, -23.9562)
  spline S463 degree 3 poles (-33.9818, -23.9562) (-33.7065, -23.9562) (-33.4815, -24.1811) (-33.4815, -24.4562) knots 6 6 6 6 7 7 7 7
  line L463 (-33.4815, -24.4562) -> (-33.4815, -37.456)
  spline S464 degree 3 poles (-138.2566, 24.4559) (-138.2566, 24.1808) (-138.4816, 23.9558) (-138.7568, 23.9558) knots 0 0 0 0 1 1 1 1
  line L464 (-138.7568, 23.9558) -> (-151.7569, 23.9558)
  spline S465 degree 3 poles (-151.7569, 23.9558) (-152.0318, 23.9558) (-152.2568, 24.1808) (-152.2568, 24.4559) knots 2 2 2 2 3 3 3 3
  line L465 (-152.2568, 24.4559) -> (-152.2568, 37.456)
  spline S466 degree 3 poles (-152.2568, 37.456) (-152.2568, 37.7311) (-152.0318, 37.956) (-151.7569, 37.956) knots 4 4 4 4 5 5 5 5
  line L466 (-151.7569, 37.956) -> (-138.7568, 37.956)
  spline S467 degree 3 poles (-138.7568, 37.956) (-138.4816, 37.956) (-138.2566, 37.7311) (-138.2566, 37.456) knots 6 6 6 6 7 7 7 7
  line L467 (-138.2566, 37.456) -> (-138.2566, 24.4559)
  spline S468 degree 3 poles (-138.2566, 43.5059) (-138.2566, 43.2308) (-138.4816, 43.0058) (-138.7568, 43.0058) knots 0 0 0 0 1 1 1 1
  line L468 (-138.7568, 43.0058) -> (-151.7569, 43.0058)
  spline S469 degree 3 poles (-151.7569, 43.0058) (-152.0318, 43.0058) (-152.2568, 43.2308) (-152.2568, 43.5059) knots 2 2 2 2 3 3 3 3
  line L469 (-152.2568, 43.5059) -> (-152.2568, 56.506)
  spline S470 degree 3 poles (-152.2568, 56.506) (-152.2568, 56.7811) (-152.0318, 57.006) (-151.7569, 57.006) knots 4 4 4 4 5 5 5 5
  line L470 (-151.7569, 57.006) -> (-138.7568, 57.006)
  spline S471 degree 3 poles (-138.7568, 57.006) (-138.4816, 57.006) (-138.2566, 56.7811) (-138.2566, 56.506) knots 6 6 6 6 7 7 7 7
  line L471 (-138.2566, 56.506) -> (-138.2566, 43.5059)
  spline S472 degree 3 poles (-119.2066, 24.4559) (-119.2066, 24.1808) (-119.4315, 23.9558) (-119.7068, 23.9558) knots 0 0 0 0 1 1 1 1
  line L472 (-119.7068, 23.9558) -> (-132.7069, 23.9558)
  spline S473 degree 3 poles (-132.7069, 23.9558) (-132.9818, 23.9558) (-133.2068, 24.1808) (-133.2068, 24.4559) knots 2 2 2 2 3 3 3 3
  line L473 (-133.2068, 24.4559) -> (-133.2068, 37.456)
  spline S474 degree 3 poles (-133.2068, 37.456) (-133.2068, 37.7311) (-132.9818, 37.956) (-132.7069, 37.956) knots 4 4 4 4 5 5 5 5
  line L474 (-132.7069, 37.956) -> (-119.7068, 37.956)
  spline S475 degree 3 poles (-119.7068, 37.956) (-119.4315, 37.956) (-119.2066, 37.7311) (-119.2066, 37.456) knots 6 6 6 6 7 7 7 7
  line L475 (-119.2066, 37.456) -> (-119.2066, 24.4559)
  spline S476 degree 3 poles (-19.1944, -56.506) (-19.1944, -56.7811) (-19.4193, -57.006) (-19.6946, -57.006) knots 0 0 0 0 1 1 1 1
  line L476 (-19.6946, -57.006) -> (-32.6947, -57.006)
  spline S477 degree 3 poles (-32.6947, -57.006) (-32.9696, -57.006) (-33.1946, -56.7811) (-33.1946, -56.506) knots 2 2 2 2 3 3 3 3
  line L477 (-33.1946, -56.506) -> (-33.1946, -43.5062)
  spline S478 degree 3 poles (-33.1946, -43.5062) (-33.1946, -43.2312) (-32.9696, -43.0062) (-32.6947, -43.0062) knots 4 4 4 4 5 5 5 5
  line L478 (-32.6947, -43.0062) -> (-19.6946, -43.0062)
  spline S479 degree 3 poles (-19.6946, -43.0062) (-19.4193, -43.0062) (-19.1944, -43.2312) (-19.1944, -43.5062) knots 6 6 6 6 7 7 7 7
  line L479 (-19.1944, -43.5062) -> (-19.1944, -56.506)
  spline S480 degree 3 poles (-14.4315, -37.456) (-14.4315, -37.7311) (-14.6565, -37.956) (-14.9317, -37.956) knots 0 0 0 0 1 1 1 1
  line L480 (-14.9317, -37.956) -> (-27.9315, -37.956)
  spline S481 degree 3 poles (-27.9315, -37.956) (-28.2064, -37.956) (-28.4314, -37.7311) (-28.4314, -37.456) knots 2 2 2 2 3 3 3 3
  line L481 (-28.4314, -37.456) -> (-28.4314, -24.4562)
  spline S482 degree 3 poles (-28.4314, -24.4562) (-28.4314, -24.1811) (-28.2064, -23.9562) (-27.9315, -23.9562) knots 4 4 4 4 5 5 5 5
  line L482 (-27.9315, -23.9562) -> (-14.9317, -23.9562)
  spline S483 degree 3 poles (-14.9317, -23.9562) (-14.6565, -23.9562) (-14.4315, -24.1811) (-14.4315, -24.4562) knots 6 6 6 6 7 7 7 7
  line L483 (-14.4315, -24.4562) -> (-14.4315, -37.456)
  spline S484 degree 3 poles (-157.3066, 43.5059) (-157.3066, 43.2308) (-157.5316, 43.0058) (-157.8068, 43.0058) knots 0 0 0 0 1 1 1 1
  line L484 (-157.8068, 43.0058) -> (-170.8069, 43.0058)
  spline S485 degree 3 poles (-170.8069, 43.0058) (-171.0818, 43.0058) (-171.3068, 43.2308) (-171.3068, 43.5059) knots 2 2 2 2 3 3 3 3
  line L485 (-171.3068, 43.5059) -> (-171.3068, 56.506)
  spline S486 degree 3 poles (-171.3068, 56.506) (-171.3068, 56.7811) (-171.0818, 57.006) (-170.8069, 57.006) knots 4 4 4 4 5 5 5 5
  line L486 (-170.8069, 57.006) -> (-157.8068, 57.006)
  spline S487 degree 3 poles (-157.8068, 57.006) (-157.5316, 57.006) (-157.3066, 56.7811) (-157.3066, 56.506) knots 6 6 6 6 7 7 7 7
  line L487 (-157.3066, 56.506) -> (-157.3066, 43.5059)
  spline S488 degree 3 poles (92.1805, -51.8062) (92.1805, -52.0813) (92.0509, -52.3062) (91.7347, -52.3062) (91.6051, -52.5312) (91.6051, -52.8063) knots 0 0 0 0 1 1 2 2 2 2
  line L488 (91.6051, -52.8063) -> (91.6051, -55.536)
  spline S489 degree 3 poles (91.6051, -55.536) (91.6051, -55.8111) (91.3802, -56.0361) (91.1049, -56.0361) knots 3 3 3 3 4 4 4 4
  line L489 (91.1049, -56.0361) -> (85.005, -56.0361)
  spline S490 degree 3 poles (85.005, -56.0361) (84.7301, -56.0361) (84.5051, -55.8111) (84.5051, -55.536) knots 5 5 5 5 6 6 6 6
  line L490 (84.5051, -55.536) -> (84.5051, -52.8063)
  spline S491 degree 3 poles (84.5051, -52.8063) (84.5051, -52.5312) (84.2802, -52.3062) (84.0049, -52.3062) knots 7 7 7 7 8 8 8 8
  line L491 (84.0049, -52.3062) -> (47.9802, -52.3062)
  spline S492 degree 3 poles (47.9802, -52.3062) (47.7053, -52.3062) (47.4803, -52.5312) (47.4803, -52.8063) knots 9 9 9 9 10 10 10 10
  line L492 (47.4803, -52.8063) -> (47.4803, -56.506)
  spline S493 degree 3 poles (47.4803, -56.506) (47.4803, -56.7811) (47.2554, -57.006) (46.9801, -57.006) knots 11 11 11 11 12 12 12 12
  line L493 (46.9801, -57.006) -> (33.98, -57.006)
  spline S494 degree 3 poles (33.98, -57.006) (33.7051, -57.006) (33.4801, -56.7811) (33.4801, -56.506) knots 13 13 13 13 14 14 14 14
  line L494 (33.4801, -56.506) -> (33.4801, -52.8063)
  spline S495 degree 3 poles (33.4801, -52.8063) (33.4801, -52.5312) (33.2552, -52.3062) (32.9799, -52.3062) knots 15 15 15 15 16 16 16 16
  line L495 (32.9799, -52.3062) -> (-3.0451, -52.3062)
  spline S496 degree 3 poles (-3.0451, -52.3062) (-3.32, -52.3062) (-3.545, -52.5312) (-3.545, -52.8063) knots 17 17 17 17 18 18 18 18
  line L496 (-3.545, -52.8063) -> (-3.545, -55.536)
  spline S497 degree 3 poles (-3.545, -55.536) (-3.545, -55.8111) (-3.77, -56.0361) (-4.0452, -56.0361) knots 19 19 19 19 20 20 20 20
  line L497 (-4.0452, -56.0361) -> (-10.1451, -56.0361)
  spline S498 degree 3 poles (-10.1451, -56.0361) (-10.42, -56.0361) (-10.645, -55.8111) (-10.645, -55.536) knots 21 21 21 21 22 22 22 22
  line L498 (-10.645, -55.536) -> (-10.645, -52.8063)
  spline S499 degree 3 poles (-10.645, -52.8063) (-10.645, -52.5312) (-10.7745, -52.3062) (-10.9323, -52.3062) (-11.0905, -52.3062) (-11.2196, -52.0813) (-11.2196, -51.8062) knots 23 23 23 23 24 24 24 25 25 25 25
  line L499 (-11.2196, -51.8062) -> (-11.2196, -50.0061)
  spline S500 degree 3 poles (-11.2196, -50.0061) (-11.2196, -49.731) (-11.0905, -49.5061) (-10.9323, -49.5061) (-10.7745, -49.5061) (-10.645, -49.2811) (-10.645, -49.006) knots 26 26 26 26 27 27 27 28 28 28 28
  line L500 (-10.645, -49.006) -> (-10.645, -43.7364)
  spline S501 degree 3 poles (-10.645, -43.7364) (-10.645, -43.4613) (-10.42, -43.2363) (-10.1451, -43.2363) knots 29 29 29 29 30 30 30 30
  line L501 (-10.1451, -43.2363) -> (-9.4203, -43.2363)
  spline S502 degree 3 poles (-9.4203, -43.2363) (-9.145, -43.2363) (-8.92, -43.0114) (-8.92, -42.7363) knots 31 31 31 31 32 32 32 32
  line L502 (-8.92, -42.7363) -> (-8.92, -42.5361)
  spline S503 degree 3 poles (-8.92, -42.5361) (-8.92, -42.261) (-8.6951, -42.036) (-8.4202, -42.036) knots 33 33 33 33 34 34 34 34
  line L503 (-8.4202, -42.036) -> (-5.7702, -42.036)
  spline S504 degree 3 poles (-5.7702, -42.036) (-5.4949, -42.036) (-5.27, -42.261) (-5.27, -42.5361) knots 35 35 35 35 36 36 36 36
  line L504 (-5.27, -42.5361) -> (-5.27, -42.7363)
  spline S505 degree 3 poles (-5.27, -42.7363) (-5.27, -43.0114) (-5.045, -43.2363) (-4.7701, -43.2363) knots 37 37 37 37 38 38 38 38
  line L505 (-4.7701, -43.2363) -> (-4.0452, -43.2363)
  spline S506 degree 3 poles (-4.0452, -43.2363) (-3.77, -43.2363) (-3.545, -43.4613) (-3.545, -43.7364) knots 39 39 39 39 40 40 40 40
  line L506 (-3.545, -43.7364) -> (-3.545, -47.2063)
  spline S507 degree 3 poles (-3.545, -47.2063) (-3.545, -47.4814) (-3.32, -47.7063) (-3.0451, -47.7063) knots 41 41 41 41 42 42 42 42
  line L507 (-3.0451, -47.7063) -> (32.9799, -47.7063)
  spline S508 degree 3 poles (32.9799, -47.7063) (33.2552, -47.7063) (33.4801, -47.4814) (33.4801, -47.2063) knots 43 43 43 43 44 44 44 44
  line L508 (33.4801, -47.2063) -> (33.4801, -43.5062)
  spline S509 degree 3 poles (33.4801, -43.5062) (33.4801, -43.2312) (33.7051, -43.0062) (33.98, -43.0062) knots 45 45 45 45 46 46 46 46
  line L509 (33.98, -43.0062) -> (46.9801, -43.0062)
  spline S510 degree 3 poles (46.9801, -43.0062) (47.2554, -43.0062) (47.4803, -43.2312) (47.4803, -43.5062) knots 47 47 47 47 48 48 48 48
  line L510 (47.4803, -43.5062) -> (47.4803, -47.2063)
  spline S511 degree 3 poles (47.4803, -47.2063) (47.4803, -47.4814) (47.7053, -47.7063) (47.9802, -47.7063) knots 49 49 49 49 50 50 50 50
  line L511 (47.9802, -47.7063) -> (84.0049, -47.7063)
  spline S512 degree 3 poles (84.0049, -47.7063) (84.2802, -47.7063) (84.5051, -47.4814) (84.5051, -47.2063) knots 51 51 51 51 52 52 52 52
  line L512 (84.5051, -47.2063) -> (84.5051, -43.7364)
  spline S513 degree 3 poles (84.5051, -43.7364) (84.5051, -43.4613) (84.7301, -43.2363) (85.005, -43.2363) knots 53 53 53 53 54 54 54 54
  line L513 (85.005, -43.2363) -> (85.7299, -43.2363)
  spline S514 degree 3 poles (85.7299, -43.2363) (86.0051, -43.2363) (86.2301, -43.0114) (86.2301, -42.7363) knots 55 55 55 55 56 56 56 56
  line L514 (86.2301, -42.7363) -> (86.2301, -42.5361)
  spline S515 degree 3 poles (86.2301, -42.5361) (86.2301, -42.261) (86.4551, -42.036) (86.73, -42.036) knots 57 57 57 57 58 58 58 58
  line L515 (86.73, -42.036) -> (89.38, -42.036)
  spline S516 degree 3 poles (89.38, -42.036) (89.6549, -42.036) (89.8798, -42.261) (89.8798, -42.5361) knots 59 59 59 59 60 60 60 60
  line L516 (89.8798, -42.5361) -> (89.8798, -42.7363)
  spline S517 degree 3 poles (89.8798, -42.7363) (89.8798, -43.0114) (90.1048, -43.2363) (90.3801, -43.2363) knots 61 61 61 61 62 62 62 62
  line L517 (90.3801, -43.2363) -> (91.1049, -43.2363)
  spline S518 degree 3 poles (91.1049, -43.2363) (91.3802, -43.2363) (91.6051, -43.4613) (91.6051, -43.7364) knots 63 63 63 63 64 64 64 64
  line L518 (91.6051, -43.7364) -> (91.6051, -49.006)
  spline S519 degree 3 poles (91.6051, -49.006) (91.6051, -49.2811) (91.7347, -49.5061) (92.0509, -49.5061) (92.1805, -49.731) (92.1805, -50.0061) knots 65 65 65 65 66 66 67 67 67 67
  line L519 (92.1805, -50.0061) -> (92.1805, -51.8062)
  spline S520 degree 3 poles (-138.2566, -37.456) (-138.2566, -37.7311) (-138.4816, -37.956) (-138.7568, -37.956) knots 0 0 0 0 1 1 1 1
  line L520 (-138.7568, -37.956) -> (-151.7569, -37.956)
  spline S521 degree 3 poles (-151.7569, -37.956) (-152.0318, -37.956) (-152.2568, -37.7311) (-152.2568, -37.456) knots 2 2 2 2 3 3 3 3
  line L521 (-152.2568, -37.456) -> (-152.2568, -24.4562)
  spline S522 degree 3 poles (-152.2568, -24.4562) (-152.2568, -24.1811) (-152.0318, -23.9562) (-151.7569, -23.9562) knots 4 4 4 4 5 5 5 5
  line L522 (-151.7569, -23.9562) -> (-138.7568, -23.9562)
  spline S523 degree 3 poles (-138.7568, -23.9562) (-138.4816, -23.9562) (-138.2566, -24.1811) (-138.2566, -24.4562) knots 6 6 6 6 7 7 7 7
  line L523 (-138.2566, -24.4562) -> (-138.2566, -37.456)
  spline S524 degree 3 poles (-57.2947, -56.506) (-57.2947, -56.7811) (-57.5197, -57.006) (-57.795, -57.006) knots 0 0 0 0 1 1 1 1
  line L524 (-57.795, -57.006) -> (-70.7947, -57.006)
  spline S525 degree 3 poles (-70.7947, -57.006) (-71.0696, -57.006) (-71.2946, -56.7811) (-71.2946, -56.506) knots 2 2 2 2 3 3 3 3
  line L525 (-71.2946, -56.506) -> (-71.2946, -43.5062)
  spline S526 degree 3 poles (-71.2946, -43.5062) (-71.2946, -43.2312) (-71.0696, -43.0062) (-70.7947, -43.0062) knots 4 4 4 4 5 5 5 5
  line L526 (-70.7947, -43.0062) -> (-57.795, -43.0062)
  spline S527 degree 3 poles (-57.795, -43.0062) (-57.5197, -43.0062) (-57.2947, -43.2312) (-57.2947, -43.5062) knots 6 6 6 6 7 7 7 7
  line L527 (-57.2947, -43.5062) -> (-57.2947, -56.506)
extrude "押し出し1" add sketch "スケッチ1" along normal blind 2 makes body 1 in component "CasePlateDefault"